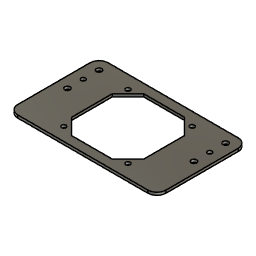
2_Base_PSU (Autodesk Fusion 360 design; units mm, degrees)
Autodesk Fusion 360 part; units mm, degrees
sketch "Sketch1" plane through (0, 0, 0) normal (0, 0, 1) x (1, 0, 0)
  line L0 (35.5, 35.5) -> (-35.5, 35.5) construction
  line L1 (-35.5, 35.5) -> (-35.5, -35.5) construction
  line L2 (-35.5, -35.5) -> (35.5, -35.5) construction
  line L3 (35.5, -35.5) -> (35.5, 35.5) construction
  line L4 (35.5, 35.5) -> (-35.5, -35.5) construction
  line L5 (-35.5, 35.5) -> (35.5, -35.5) construction
  circle A0 centre (-35.5, 35.5) radius 2.5
  circle A1 centre (35.5, 35.5) radius 2.5
  circle A2 centre (-35.5, -35.5) radius 2.5
  circle A3 centre (35.5, -35.5) radius 2.5
  line L6 (63, 50) -> (-63, 50) construction
  line L7 (-63, 50) -> (-63, -50) construction
  line L8 (-63, -50) -> (63, -50) construction
  line L9 (63, -50) -> (63, 50) construction
  line L10 (63, 50) -> (-63, -50) construction
  line L11 (-63, 50) -> (63, -50) construction
  line L12 (40, 40) -> (-40, 40) construction
  line L13 (-40, 40) -> (-40, -40) construction
  line L14 (-40, -40) -> (40, -40) construction
  line L15 (40, -40) -> (40, 40) construction
  line L16 (40, 40) -> (-40, -40) construction
  line L17 (-40, 40) -> (40, -40) construction
  line L18 (-22.5, 40) -> (-40, 22.5)
  line L19 (0, 0) -> (0, 35.5) construction
  line L20 (0, 0) -> (35.5, 0) construction
  line L21 (22.5, 40) -> (40, 22.5)
  line L22 (-22.5, -40) -> (-40, -22.5)
  line L23 (22.5, -40) -> (40, -22.5)
  line L24 (-40, -22.5) -> (-40, 22.5)
  line L25 (-22.5, 40) -> (22.5, 40)
  line L26 (40, 22.5) -> (40, -22.5)
  line L27 (-22.5, -40) -> (22.5, -40)
  circle A4 centre (-70, 3) radius 3
  circle A5 centre (-70, 38) radius 3
  circle A6 centre (70, 38) radius 3
  circle A7 centre (70, 3) radius 3
  line L28 (-70, 38) -> (-70, 3) construction
  circle A8 centre (-70, 20.5) radius 2.5
  circle A9 centre (70, 20.5) radius 2.5
  line L29 (-72, -50) -> (72, -50)
  line L30 (82, -40) -> (82, 40)
  line L31 (72, 50) -> (-72, 50)
  line L32 (-82, 40) -> (-82, -40)
  arc A10 (-72, 50) -> (-82, 40) centre (-72, 40) ccw
  arc A11 (82, 40) -> (72, 50) centre (72, 40) ccw
  arc A12 (72, -50) -> (82, -40) centre (72, -40) ccw
  arc A13 (-82, -40) -> (-72, -50) centre (-72, -40) ccw
  point P0 (-70, 38)
  point P1 (-82, -50)
  point P2 (82, -50)
  point P3 (82, 50)
  dimension "d1" = 71
  dimension "d2" = 71
  dimension "d3" = 5
  dimension "d4" = 5
  dimension "d5" = 5
  dimension "d6" = 5
  dimension "d7" = 126
  dimension "d8" = 100
  dimension "d9" = 80
  dimension "d10" = 80
  dimension "d11" = 13
  dimension "d12" = 45
  dimension "d13" = 12
  dimension "d14" = 70
  dimension "d15" = 5
  dimension "d16" = 12
  dimension "d17" = 10
  constraint horizontal L0
  constraint perpendicular L0 L1
  constraint parallel L0 L2
  constraint parallel L1 L3
  constraint coincident L4 L19.start
  constraint coincident L5 L19.start
  constraint coincident L19.start L20.start
  constraint coincident L0.end L1.start
  constraint coincident L0.start L3.end
  constraint coincident L1.end L2.start
  constraint coincident L2.end L3.start
  constraint horizontal L6
  constraint perpendicular L6 L7
  constraint parallel L6 L8
  constraint parallel L7 L9
  constraint coincident L10 L19.start
  constraint coincident L11 L19.start
  constraint horizontal L12
  constraint perpendicular L12 L13
  constraint parallel L12 L14
  constraint parallel L13 L15
  constraint coincident L16 L19.start
  constraint coincident L17 L19.start
  constraint coincident L12 L18.start
  constraint coincident L13 L18.end
  constraint midpoint L0 L19.end
  constraint midpoint L3 L20.end
  constraint symmetric L18.start L19 L21.start
  constraint symmetric L18.end L19 L21.end
  constraint symmetric L18.start L20 L22.start
  constraint symmetric L18.end L20 L22.end
  constraint symmetric L20 L21.start L23.start
  constraint symmetric L20 L21.end L23.end
  constraint coincident P0 A5.centre
  constraint coincident A4.centre L28.end
  constraint midpoint L28 A8.centre
  constraint symmetric L19 A8 A9
  constraint horizontal L7.end P1
  constraint symmetric L19 P1 P2
  constraint symmetric L20 P2 P3
  constraint horizontal L29
  constraint vertical L30
  constraint horizontal L31
  constraint vertical L32
  constraint tangent L32 A10
  constraint tangent L31 A10
  constraint tangent L30 A11
  constraint tangent L31 A11
  constraint equal A10 A11
  constraint tangent L30 A12
  constraint tangent L29 A12
  constraint equal A10 A12
  constraint tangent L29 A13
  constraint tangent L32 A13
  constraint equal A10 A13
  measures "d1" distance of L1.end L2.end
  measures "d2" distance of L0.end L1.end
  measures "d3" diameter of A0
  measures "d4" diameter of A1
  measures "d5" diameter of A2
  measures "d6" diameter of A3
  measures "d7" distance of L7.end L8.end
  measures "d8" distance of L6.end L7.end
  measures "d9" distance of L13.end L14.end
  measures "d10" distance of L12.end L13.end
  measures "d11" horizontal distance of L0.end L18.start
  measures "d12" angle of L12 L18
  measures "d13" distance of L6 P0
  measures "d14" horizontal distance of L19.start A5.centre
  measures "d15" diameter of A8
  measures "d16" horizontal distance of A4.centre P1
  measures "d17" radius of A10
extrude "Extrude1" add sketch "Sketch1" along normal blind 3
